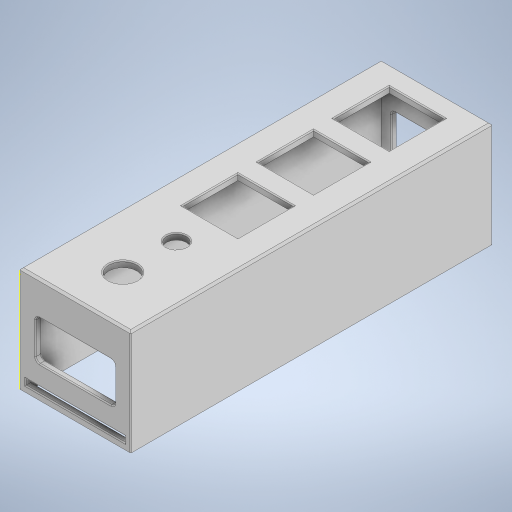
# Autodesk Inventor part: eceFinal_v1
Saved by Autodesk Inventor 2024 (Build 280153000, 153)
## iProperties
Created: 2025-11-21
Part Number: eceFinal_v1
Material: Generic
Document SubType Name: Modeling
Designer: dearl
Density: 1 g/cm^3
Appearance: Default
Author: dearl
Autodesk Inventor part; units mm, degrees
ref_plane "YZ Plane" through (0, 0, 0) normal (1, 0, 0) x (0, 1, 0)
ref_plane "XZ Plane" through (0, 0, 0) normal (0, 1, 0) x (-1, 0, 0)
ref_plane "XY Plane" through (0, 0, 0) normal (0, 0, 1) x (1, 0, 0)
sketch "Sketch1" plane through (0, 0, 0) normal (0, 1, 0) x (-1, 0, 0)
  circle A0 centre (14, -12) radius 3.55
  line L0 (7, -34) -> (21, -34)
  line L1 (21, -34) -> (21, -48)
  line L2 (21, -48) -> (7, -48)
  line L3 (7, -48) -> (7, -34)
  line L4 (7, -53.05) -> (21, -53.05)
  line L5 (21, -53.05) -> (21, -67.05)
  line L6 (21, -67.05) -> (7, -67.05)
  line L7 (7, -67.05) -> (7, -53.05)
  line L8 (7, -72.1) -> (21, -72.1)
  line L9 (21, -72.1) -> (21, -86.1)
  line L10 (21, -86.1) -> (7, -86.1)
  line L11 (7, -86.1) -> (7, -72.1)
  circle A1 centre (14, -12) radius 7
  line L12 (28, -86.1) -> (28, -91.1)
  line L13 (28, -91.1) -> (21, -91.1)
  line L14 (28, -91.1) -> (0, -91.1)
  line L15 (0, -91.1) -> (0, 0)
  line L16 (0, 0) -> (28, 0)
  line L17 (28, 0) -> (28, -91.1)
  circle A2 centre (14, -25.5) radius 2.5
  line L18 (11.5, -23) -> (16.5, -28) construction
  line L19 (16.5, -23) -> (11.5, -28) construction
  point P0 (14, 0)
  dimension "d0" = 7.1
  dimension "d1" = 14
  dimension "d2" = 14
  dimension "d5" = 19.05
  dimension "d12" = 14
  dimension "d16" = 5
  dimension "d18" = 7
  dimension "d23" = 5
  dimension "d28" = 91.1
  dimension "d29" = 28
  dimension "d30" = 14
  dimension "d32" = 14
  dimension "d33" = 13.5
  dimension "d42" = 12
  dimension "d43" = 8.5
  constraints: 40 end point, 4 parallel, 3 centre point, 3 midpoint, 3 perpendicular, 2 horizontal, 2 vertical, 1 coincident, 1 collinear, 15 other
  measures "d0" diameter of A0
  measures "d1" distance of L1.end L2.end
  measures "d2" distance of L0.end L1.end
  measures "d5" distance of L0.start L4.start
  measures "d12" diameter of A1
  measures "d16" distance of L9.end L13.end
  measures "d18" distance between parallel lines of L15 L11
  measures "d23" diameter of A2
  measures "d28" distance of L16.end L12.end
  measures "d29" distance of L12.end L14.end
  measures "d30" distance from line of L15 A2.centre
  measures "d32" distance from line of L15 A0.centre
  measures "d33" distance of A2.centre A0.centre
  measures "d42" distance of point (14, 0) A1.centre
  measures "d43" distance from line of L0 A2.centre
extrude "Extrusion1" add sketch "Sketch1" along normal blind 1.5 contours A1 | L12 L13 L14 L15 L16 L17
sketch "Sketch2" plane through (0, 1.5, 0) normal (0, 1, 0) x (1, 0, 0)
  line L0 (-7, 48) -> (-7, 34) projected
  line L1 (-21, 48) -> (-7, 48) projected
  line L2 (-7, 34) -> (-21, 48)
  line L3 (-23, 32) -> (-5, 32)
  line L4 (-5, 32) -> (-5, 50)
  line L5 (-5, 50) -> (-23, 50)
  line L6 (-23, 50) -> (-23, 32)
  line L7 (-23, 32) -> (-5, 50) construction
  line L8 (-5, 32) -> (-23, 50) construction
  line L9 (-7, 67.05) -> (-7, 53.05) projected
  line L10 (-21, 67.05) -> (-7, 67.05) projected
  line L11 (-7, 53.05) -> (-21, 67.05)
  line L12 (-23, 51.05) -> (-5, 51.05)
  line L13 (-5, 51.05) -> (-5, 69.05)
  line L14 (-5, 69.05) -> (-23, 69.05)
  line L15 (-23, 69.05) -> (-23, 51.05)
  line L16 (-23, 51.05) -> (-5, 69.05) construction
  line L17 (-5, 51.05) -> (-23, 69.05) construction
  line L18 (-7, 72.1) -> (-21, 72.1) projected
  line L19 (-21, 72.1) -> (-21, 86.1) projected
  line L20 (-7, 72.1) -> (-21, 86.1)
  line L21 (-23, 70.1) -> (-5, 70.1)
  line L22 (-5, 70.1) -> (-5, 88.1)
  line L23 (-5, 88.1) -> (-23, 88.1)
  line L24 (-23, 88.1) -> (-23, 70.1)
  line L25 (-23, 70.1) -> (-5, 88.1) construction
  line L26 (-5, 70.1) -> (-23, 88.1) construction
  circle A0 centre (-14, 12) radius 3.55 projected
  circle A1 centre (-14, 12) radius 7
  line L27 (-7, 34) -> (-21, 34) projected
  line L28 (-14, 19) -> (-14, 25.5)
  point P0 (0, 0)
  point P1 (-14, 41)
  point P2 (-14, 60.05)
  point P3 (-14, 79.1)
  dimension "d38" = 14
  dimension "d34" = 18
  dimension "d35" = 18
  dimension "d36" = 18
  dimension "d37" = 18
  dimension "d39" = 13
  dimension "d41" = 6.5
  constraints: 44 end point, 9 midpoint, 6 parallel, 3 horizontal, 3 perpendicular, 2 coincident, 1 vertical, 1 vertical alignment, 2 other
  measures "d34" distance of L5.end L4.end
  measures "d35" distance of L13.end L12.end
  measures "d36" distance of L23.end L22.end
  measures "d37" distance of L22.end L21.end
  measures "d41" distance of L28.start L28.end
sketch "Sketch3" plane through (0, 0, 0) normal (0, -1, 0) x (1, 0, 0)
  line L0 (-28, 0) -> (0, 0) projected
  line L1 (0, -91.1) -> (-28, -91.1) projected
  line L2 (0, 0) -> (-28, 0)
  line L3 (-28, 0) -> (-28, -91.1)
  line L4 (-28, -91.1) -> (0, -91.1)
  line L5 (0, -91.1) -> (0, 0)
  line L6 (-1.5, -1.5) -> (-26.5, -1.5)
  line L7 (-26.5, -1.5) -> (-26.5, -89.6)
  line L8 (-26.5, -89.6) -> (-1.5, -89.6)
  line L9 (-1.5, -89.6) -> (-1.5, -1.5)
  dimension "d44" = 1.5
  constraints: 16 end point, 4 parallel, 2 perpendicular, 1 horizontal, 3 other
  measures "d44" distance between parallel lines of L5 L9
extrude "Extrusion2" add sketch "Sketch3" along normal blind 25
chamfer "Chamfer1" distance 0.5 angle 45 4 edges at (-14, 1.5, 0) (-28, 1.5, -45.55) (-14, 1.5, -91.1) (0, 1.5, -45.55)
fillet "Fillet1" radius 0.25 1 edges at (-10.45, 1.5, -12)
fillet "Fillet2" radius 0.25 1 edges at (-11.5, 1.5, -25.5)
fillet "Fillet3" radius 0.25 12 edges at (-14, 1.5, -34) (-21, 1.5, -41) (-14, 1.5, -48) (-7, 1.5, -41) (-14, 1.5, -53.05) (-21, 1.5, -60.05) (-14, 1.5, -67.05) (-7, 1.5, -60.05) (-14, 1.5, -72.1) (-21, 1.5, -79.1) (-14, 1.5, -86.1) (-7, 1.5, -79.1)
sketch "Sketch4" plane through (-28, -25, 0) normal (0, 0, 1) x (1, 0, 0)
  line L0 (0.5, 26.5) -> (0, 26) projected
  line L1 (28, 0) -> (28, 26) projected
  line L2 (0, 26) -> (28, 0)
  line L3 (5, 8) -> (23, 8)
  line L4 (24, 9) -> (24, 17)
  line L5 (23, 18) -> (5, 18)
  line L6 (4, 17) -> (4, 9)
  line L7 (4, 8) -> (24, 18) construction
  line L8 (24, 8) -> (4, 18) construction
  arc A0 (5, 18) -> (4, 17) centre (5, 17) ccw
  arc A1 (4, 9) -> (5, 8) centre (5, 9) ccw
  arc A2 (23, 8) -> (24, 9) centre (23, 9) ccw
  arc A3 (24, 17) -> (23, 18) centre (23, 17) ccw
  point P0 (28, 25)
  point P1 (14, 13)
  dimension "d53" = 20
  dimension "d54" = 10
  dimension "d55" = 1
  dimension "d56" = 1
  constraints: 14 end point, 8 point on circle, 8 point on line, 8 tangent, 4 centre point, 3 midpoint, 2 equal radius, 2 parallel, 1 horizontal, 1 perpendicular
  measures "d53" distance of L8.end L7.end
  measures "d54" distance of L7.end L8.start
  measures "d55" radius of A0
  measures "d56" radius of A1
extrude "Extrusion3" cut sketch "Sketch4" against normal through all
fillet "Fillet4" radius 0.25 32 edges at (-23.7071, -7.2929, -91.1) (-24, -12, -91.1) (-23.7071, -16.7071, -91.1) (-14, -17, -91.1) (-4.2929, -16.7071, -91.1) (-4, -12, -91.1) (-4.2929, -7.2929, -91.1) (-14, -7, -91.1) (-4.2929, -7.2929, -89.6) (-4, -12, -89.6) (-4.2929, -16.7071, -89.6) (-14, -17, -89.6) (-23.7071, -16.7071, -89.6) (-24, -12, -89.6) (-23.7071, -7.2929, -89.6) (-14, -7, -89.6) (-4.2929, -7.2929, -1.5) (-14, -7, -1.5) (-23.7071, -7.2929, -1.5) (-24, -12, -1.5) (-23.7071, -16.7071, -1.5) (-14, -17, -1.5) (-4.2929, -16.7071, -1.5) (-4, -12, -1.5) (-4.2929, -16.7071, 0) (-14, -17, 0) (-23.7071, -16.7071, 0) (-24, -12, 0) (-23.7071, -7.2929, 0) (-14, -7, 0) (-4.2929, -7.2929, 0) (-4, -12, 0)
fillet "Fillet5" radius 0.25 4 edges at (-28, -12, -91.1) (0, -12, -91.1) (-28, -12, 0) (0, -12, 0)
sketch "Sketch5" plane through (-0.25, -25, -91.1) normal (0, 0, -1) x (-1, 0, 0)
  line L0 (0, 0) -> (-0.25, 0) projected
  line L1 (-0.25, 0) -> (1.25, 0)
  line L2 (1.25, 0) -> (1.25, 3)
  line L3 (1.25, 3) -> (-0.25, 3)
  line L4 (-0.25, 3) -> (-0.25, 0)
  line L5 (27.75, 26) -> (27.75, 0) projected
  line L6 (27.75, 0) -> (26.25, 0)
  line L7 (26.25, 0) -> (26.25, 3)
  line L8 (26.25, 3) -> (27.75, 3)
  line L9 (27.75, 3) -> (27.75, 0)
  line L10 (1.25, 3) -> (26.25, 3)
  line L11 (26.25, 3) -> (26.25, 1.5)
  line L12 (26.25, 1.5) -> (1.25, 1.5)
  line L13 (1.25, 1.5) -> (1.25, 3)
  point P0 (-0.25, 25)
  dimension "d61" = 1.5
  dimension "d62" = 3
  dimension "d63" = 1.5
  dimension "d64" = 3
  dimension "d65" = 1.5
  constraints: 24 end point, 6 parallel, 3 horizontal, 3 perpendicular, 1 midpoint
  measures "d61" distance of L3.end L2.end
  measures "d62" distance of L2.end L1.end
  measures "d63" distance of L7.end L8.end
  measures "d64" distance of L6.end L7.end
  measures "d65" distance of L10.end L11.end
extrude "Extrusion4" cut sketch "Sketch5" against normal through all contours L2 L10 L7 L12
fillet "Fillet6" radius 0.25 12 edges at (-14, -22, -91.1) (-26.5, -22.75, -91.1) (-14, -23.5, -91.1) (-1.5, -22.75, -91.1) (-14, -23.5, -89.6) (-14, -22, -89.6) (-1.5, -22.75, 0) (-14, -22, 0) (-14, -23.5, 0) (-26.5, -22.75, 0) (-14, -22, -1.5) (-14, -23.5, -1.5)
sketch "Sketch6" plane through (-28, -25, -0.25) normal (-1, 0, 0) x (0, 0, 1)
  line L0 (0.25, 0) -> (0.25, 26) projected
  line L1 (-90.85, 26) -> (-90.85, 0) projected
  point P0 (0.25, 25)
body "Solid1"
